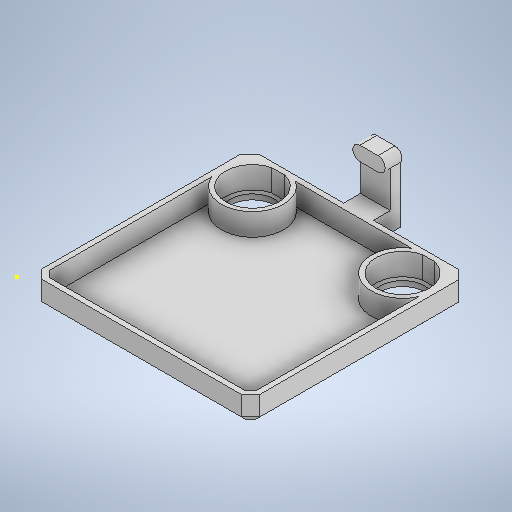
# Autodesk Inventor part: case_v1.4_b
Saved by Autodesk Inventor 2025 (Build 290162000, 162)
## iProperties
Created: 2025-03-20
Part Number: case_v1.4_b
Material: Generic
Document SubType Name: Modeling
Designer: ethan
Density: 1 g/cm^3
Appearance: Default
Author: ethan
Autodesk Inventor part; units mm, degrees
ref_plane "YZ Plane" through (0, 0, 0) normal (1, 0, 0) x (0, 1, 0)
ref_plane "XZ Plane" through (0, 0, 0) normal (0, 1, 0) x (-1, 0, 0)
ref_plane "XY Plane" through (0, 0, 0) normal (0, 0, 1) x (1, 0, 0)
sketch "Sketch1" plane through (0, 0, 0) normal (0, 1, 0) x (-1, 0, 0)
  line L0 (0, 0) -> (-88, 0)
  line L1 (-88, 0) -> (-88, -94)
  line L2 (-88, -94) -> (0, -94)
  line L3 (0, -94) -> (0, 0)
  line L4 (0, -94) -> (0, -75.65)
  line L5 (0, -94) -> (-15.05, -94)
  circle A0 centre (-15.05, -75.65) radius 8.5
  line L6 (-44, -88.9444) -> (-44, -54.2543) construction
  circle A1 centre (-72.95, -75.65) radius 8.5
  line L7 (-15.05, -94) -> (-15.05, -77.2221)
  line L8 (-15.05, -77.2221) -> (-15.05, -73.1555)
  dimension "d0" = 88
  dimension "d1" = 94
  dimension "d2" = 18.35
  dimension "d3" = 15.05
  dimension "d4" = 17
  dimension "d48" = 17
  constraints: 18 end point, 3 point on line, 3 vertical, 2 centre point, 2 parallel, 1 horizontal, 1 perpendicular, 1 symmetric about line, 1 other
  measures "d0" distance of L2.end L1.end
  measures "d1" distance of L1.end L0.end
  measures "d2" distance of L2.end L4.end
  measures "d3" distance of L2.end L5.end
  measures "d4" diameter of A0
  measures "d48" diameter of A1
extrude "Extrusion1" add sketch "Sketch1" along normal blind 2
sketch "Sketch3" plane through (0, 2, 0) normal (0, 1, 0) x (1, 0, 0)
  circle A0 centre (72.95, 75.65) radius 8.5 construction
  circle A1 centre (15.05, 75.65) radius 8.5 construction
  line L0 (0, 0) -> (4, 0) construction
  line L1 (4, 0) -> (4, 6) construction
  line L2 (4, 6) -> (0, 6) construction
  line L3 (0, 6) -> (0, 0) construction
  line L4 (88, 0) -> (84, 0) construction
  line L5 (84, 0) -> (84, 6) construction
  line L6 (84, 6) -> (88, 6) construction
  line L7 (88, 6) -> (88, 0) construction
  line L8 (4, 6) -> (2, 6) construction
  line L9 (2, 6) -> (2, 4) construction
  line L10 (2, 4) -> (4, 4) construction
  line L11 (4, 4) -> (4, 6) construction
  line L12 (2, 4) -> (6, 4)
  line L13 (6, 4) -> (6, 6)
  line L14 (6, 6) -> (2, 6)
  line L15 (2, 6) -> (2, 4)
  line L16 (2, 4) -> (4, 4)
  line L17 (4, 4) -> (4, 8)
  line L18 (4, 8) -> (2, 8)
  line L19 (2, 8) -> (2, 4)
  line L20 (86, 4) -> (82, 4)
  line L21 (82, 4) -> (82, 4)
  line L22 (82, 4) -> (86, 4)
  line L23 (86, 4) -> (86, 4)
  line L24 (86, 4) -> (84, 4)
  line L25 (84, 4) -> (84, 8)
  line L26 (84, 8) -> (86, 8)
  line L27 (86, 8) -> (86, 4)
  line L28 (44, 4.3599) -> (37, 4.3599) construction
  line L29 (88, -1) -> (0, -1) construction
  line L30 (37, -1) -> (51, -1) construction
  line L31 (51, -1) -> (51, 0) construction
  line L32 (51, 0) -> (37, 0) construction
  line L33 (37, 0) -> (37, -1) construction
  line L34 (37, -1) -> (51, -1)
  line L35 (51, -1) -> (51, 0)
  line L36 (51, 0) -> (37, 0)
  line L37 (37, 0) -> (37, -1)
  line L38 (0, 95) -> (88, 95) projected
  line L39 (37, 95) -> (51, 95)
  line L40 (51, 95) -> (51, 94)
  line L41 (51, 94) -> (37, 94)
  line L42 (37, 94) -> (37, 95)
  circle A2 centre (15.05, 75.65) radius 10.5
  circle A3 centre (15.05, 75.65) radius 12
  line L43 (15.05, 75.65) -> (27.05, 75.65) construction
  line L44 (15.05, 75.65) -> (21.05, 86.0423) construction
  line L45 (15.05, 75.65) -> (9.05, 86.0423) construction
  line L46 (15.05, 75.65) -> (3.05, 75.65) construction
  line L47 (15.05, 75.65) -> (9.05, 65.2577) construction
  line L48 (15.05, 75.65) -> (21.05, 65.2577) construction
  line L49 (9.8, 84.7433) -> (9.05, 86.0423) construction
  line L50 (9.8, 84.7433) -> (9.05, 86.0423)
  line L51 (21.05, 86.0423) -> (20.3, 84.7433)
  line L52 (25.55, 75.65) -> (27.05, 75.65)
  line L53 (21.05, 65.2577) -> (20.3, 66.5567)
  line L54 (9.8, 66.5567) -> (9.05, 65.2577)
  line L55 (4.55, 75.65) -> (3.05, 75.65)
  line L56 (44, 84.7433) -> (44, 74.6259) construction
  circle A4 centre (72.95, 75.65) radius 8.5 construction
  circle A5 centre (72.95, 75.65) radius 10.5
  circle A6 centre (72.95, 75.65) radius 12
  line L57 (72.95, 75.65) -> (60.95, 75.65) construction
  line L58 (72.95, 75.65) -> (66.95, 86.0423) construction
  line L59 (72.95, 75.65) -> (78.95, 86.0423) construction
  line L60 (72.95, 75.65) -> (84.95, 75.65) construction
  line L61 (72.95, 75.65) -> (78.95, 65.2577) construction
  line L62 (72.95, 75.65) -> (66.95, 65.2577) construction
  line L63 (78.2, 84.7433) -> (78.95, 86.0423) construction
  line L64 (78.2, 84.7433) -> (78.95, 86.0423)
  line L65 (66.95, 86.0423) -> (67.7, 84.7433)
  line L66 (62.45, 75.65) -> (60.95, 75.65)
  line L67 (66.95, 65.2577) -> (67.7, 66.5567)
  line L68 (78.2, 66.5567) -> (78.95, 65.2577)
  line L69 (83.45, 75.65) -> (84.95, 75.65)
  line L70 (86, 4) -> (82, 4)
  line L71 (82, 4) -> (82, 6)
  line L72 (82, 6) -> (86, 6)
  line L73 (86, 6) -> (86, 4)
  point P0 (2, 4)
  point P1 (4, 6)
  point P2 (84, 4)
  point P3 (84.95, 75.65)
  point P4 (78.95, 65.2577)
  point P5 (3.05, 75.65)
  point P6 (9.05, 65.2577)
  point P7 (84, 6)
  dimension "d11" = 4
  dimension "d12" = 6
  dimension "d13" = 4
  dimension "d14" = 6
  dimension "d15" = 2
  dimension "d16" = 2
  dimension "d17" = 4
  dimension "d18" = 4
  dimension "d19" = 4
  dimension "d20" = 2
  dimension "d21" = 4
  dimension "d22" = 7
  dimension "d23" = 14
  dimension "d24" = 14
  dimension "d25" = 1
  dimension "d26" = 2
  dimension "d27" = 1.5
  dimension "d30" = 360
  constraints: 144 end point, 21 parallel, 19 symmetric about line, 17 point on line, 16 point on circle, 11 perpendicular, 10 horizontal, 7 collinear, 5 centre point, 2 coincident, 1 vertical, 20 other
  measures "d11" distance of L2.end L1.end
  measures "d12" distance of L1.end L0.end
  measures "d13" distance of L5.end L6.end
  measures "d14" distance of L4.end L5.end
  measures "d15" distance of L10.end L9.end
  measures "d16" distance of L9.end L8.end
  measures "d17" distance of L14.end L13.end
  measures "d18" distance of L17.end L16.end
  measures "d19" distance of L21.end L22.end
  measures "d20" distance of L25.end L26.end
  measures "d21" distance of L24.end L25.end
  measures "d22" distance of L28.start L28.end
  measures "d23" distance of L30.start L30.end
  measures "d24" distance of L39.start L39.end
  measures "d25" distance of L39.end L40.end
  measures "d26" radial gap between concentric circles of A1 A2
  measures "d27" radial gap between concentric circles of A2 A3
extrude "Extrusion3" add sketch "Sketch3" along normal blind 8.5 contours L52 A3 L53 A2 | A2 L50 A3 L51 | L54 A3 L55 A2 | L69 A6 L68 A5 | A5 L65 A6 L64 | L67 A6 L66 A5
sketch "Sketch7" plane through (0, 2, 0) normal (0, 1, 0) x (1, 0, 0)
  line L0 (3.05, 75.65) -> (4.55, 75.65) construction
  arc A0 (4.55, 75.65) -> (9.8, 66.5567) centre (15.05, 75.65) ccw construction
  line L1 (9.8, 66.5567) -> (9.05, 65.2577) construction
  arc A1 (3.05, 75.65) -> (9.05, 65.2577) centre (15.05, 75.65) ccw construction
  arc A2 (78.95, 65.2577) -> (84.95, 75.65) centre (72.95, 75.65) ccw construction
  line L2 (78.95, 65.2577) -> (78.2, 66.5567) construction
  arc A3 (78.2, 66.5567) -> (83.45, 75.65) centre (72.95, 75.65) ccw construction
  line L3 (83.45, 75.65) -> (84.95, 75.65) construction
  arc A4 (78.2, 84.7433) -> (67.7, 84.7433) centre (72.95, 75.65) ccw construction
  line L4 (67.7, 84.7433) -> (66.95, 86.0423) construction
  arc A5 (78.95, 86.0423) -> (66.95, 86.0423) centre (72.95, 75.65) ccw construction
  line L5 (78.95, 86.0423) -> (78.2, 84.7433) construction
  line L6 (21.05, 86.0423) -> (20.3, 84.7433) construction
  arc A6 (20.3, 84.7433) -> (9.8, 84.7433) centre (15.05, 75.65) ccw construction
  line L7 (9.8, 84.7433) -> (9.05, 86.0423) construction
  arc A7 (21.05, 86.0423) -> (9.05, 86.0423) centre (15.05, 75.65) ccw construction
  arc A8 (62.45, 75.65) -> (67.7, 66.5567) centre (72.95, 75.65) ccw construction
  line L8 (67.7, 66.5567) -> (66.95, 65.2577) construction
  arc A9 (60.95, 75.65) -> (66.95, 65.2577) centre (72.95, 75.65) ccw construction
  line L9 (60.95, 75.65) -> (62.45, 75.65) construction
  line L10 (25.55, 75.65) -> (27.05, 75.65) construction
  arc A10 (21.05, 65.2577) -> (27.05, 75.65) centre (15.05, 75.65) ccw construction
  line L11 (21.05, 65.2577) -> (20.3, 66.5567) construction
  arc A11 (20.3, 66.5567) -> (25.55, 75.65) centre (15.05, 75.65) ccw construction
  line L12 (88, 94) -> (0, 94) construction
  line L13 (0, 94) -> (0, 0) construction
  line L14 (0, 0) -> (88, 0) construction
  line L15 (88, 0) -> (88, 94) construction
  circle A12 centre (72.95, 75.65) radius 8.5 construction
  circle A13 centre (15.05, 75.65) radius 8.5 construction
  line L16 (2, 4) -> (86, 4) construction
  line L17 (86, 4) -> (86, 94) construction
  line L18 (86, 94) -> (2, 94) construction
  line L19 (2, 94) -> (2, 4) construction
  line L20 (0, 0) -> (88, 0)
  line L21 (88, 0) -> (88, 94)
  line L22 (88, 94) -> (0, 94)
  line L23 (0, 94) -> (0, 0)
  line L24 (86, 94) -> (2, 94)
  line L25 (2, 94) -> (2, 4)
  line L26 (2, 4) -> (86, 4)
  line L27 (86, 4) -> (86, 94)
  point P0 (2, 94)
  constraints: 24 end point, 6 parallel, 3 horizontal, 3 perpendicular, 1 point on line
extrude "Extrusion7" cut sketch "Sketch7" against normal up to surface (2 mm away) contours L23 L22 L25 L26 L27 L21 L20
sketch "Sketch8" plane through (0, 2, 0) normal (0, 1, 0) x (1, 0, 0)
  circle A0 centre (15.05, 75.65) radius 8.5 projected
  circle A1 centre (72.95, 75.65) radius 8.5 projected
  line L0 (86, 4) -> (86, 94) projected
  line L1 (86, 94) -> (2, 94) projected
  line L2 (2, 94) -> (2, 4) projected
  line L3 (3.05, 75.65) -> (4.55, 75.65) projected
  arc A2 (4.55, 75.65) -> (9.8, 66.5567) centre (15.05, 75.65) ccw projected
  line L4 (9.8, 66.5567) -> (9.05, 65.2577) projected
  arc A3 (3.05, 75.65) -> (9.05, 65.2577) centre (15.05, 75.65) ccw projected
  arc A4 (78.95, 65.2577) -> (84.95, 75.65) centre (72.95, 75.65) ccw projected
  line L5 (78.95, 65.2577) -> (78.2, 66.5567) projected
  arc A5 (78.2, 66.5567) -> (83.45, 75.65) centre (72.95, 75.65) ccw projected
  line L6 (83.45, 75.65) -> (84.95, 75.65) projected
  line L7 (25.55, 75.65) -> (27.05, 75.65) projected
  arc A6 (21.05, 65.2577) -> (27.05, 75.65) centre (15.05, 75.65) ccw projected
  line L8 (21.05, 65.2577) -> (20.3, 66.5567) projected
  arc A7 (20.3, 66.5567) -> (25.55, 75.65) centre (15.05, 75.65) ccw projected
  arc A8 (62.45, 75.65) -> (67.7, 66.5567) centre (72.95, 75.65) ccw projected
  line L9 (67.7, 66.5567) -> (66.95, 65.2577) projected
  arc A9 (60.95, 75.65) -> (66.95, 65.2577) centre (72.95, 75.65) ccw projected
  line L10 (60.95, 75.65) -> (62.45, 75.65) projected
  line L11 (21.05, 86.0423) -> (20.3, 84.7433) projected
  arc A10 (20.3, 84.7433) -> (9.8, 84.7433) centre (15.05, 75.65) ccw projected
  line L12 (9.8, 84.7433) -> (9.05, 86.0423) projected
  arc A11 (21.05, 86.0423) -> (9.05, 86.0423) centre (15.05, 75.65) ccw projected
  arc A12 (78.2, 84.7433) -> (67.7, 84.7433) centre (72.95, 75.65) ccw projected
  line L13 (67.7, 84.7433) -> (66.95, 86.0423) projected
  arc A13 (78.95, 86.0423) -> (66.95, 86.0423) centre (72.95, 75.65) ccw projected
  line L14 (78.95, 86.0423) -> (78.2, 84.7433) projected
  line L15 (86, 4) -> (2, 4) projected
  line L16 (2, 75.65) -> (86, 75.65)
  line L17 (86, 75.65) -> (86, 7.5)
  line L18 (82.5, 4) -> (5.5, 4)
  line L19 (2, 7.5) -> (2, 75.65)
  line L20 (2, 7.5) -> (5.5, 4)
  line L21 (82.5, 4) -> (86, 7.5)
  line L22 (4, 73.65) -> (84, 73.65)
  line L23 (84, 73.65) -> (84, 8.3284)
  line L24 (84, 8.3284) -> (81.6716, 6)
  line L25 (81.6716, 6) -> (6.3284, 6)
  line L26 (6.3284, 6) -> (4, 8.3284)
  line L27 (4, 8.3284) -> (4, 73.65)
  line L28 (2, 4) -> (86, 4) projected
  point P0 (0, 0)
  point P1 (2, 4)
  point P2 (4, 70.9705)
  point P3 (3.05, 75.65)
  point P4 (5.5, 4)
  point P5 (84.95, 75.65)
  point P6 (84, 70.9705)
  dimension "d51" = 3.5
  dimension "d52" = 3.5
  dimension "d53" = 3.5
  dimension "d54" = 3.5
  dimension "d55" = 2
  constraints: 24 end point, 4 parallel, 4 point on line, 2 perpendicular, 1 horizontal, 5 other
  measures "d51" distance of L19.start point (2, 4)
  measures "d52" distance of L18.end point (2, 4)
  measures "d53" distance of L18.start L15.start
  measures "d54" distance of L17.end L15.start
  measures "d55" distance between parallel lines of L19 L27
extrude "Extrusion8" add sketch "Sketch8" along normal blind 8.5 contours A3 L27 L26 L25 L24 L23 A4 L16 L0 L21 L15 L20 L2
sketch "Sketch9" plane through (0, 2, 0) normal (0, 1, 0) x (1, 0, 0)
  line L0 (5.5, 4) -> (2, 7.5) projected
  line L1 (2, 7.5) -> (2, 4) projected
  line L2 (2, 4) -> (5.5, 4) projected
  line L3 (86, 4) -> (86, 7.5) projected
  line L4 (86, 7.5) -> (82.5, 4) projected
  line L5 (82.5, 4) -> (86, 4) projected
  line L6 (86, 4) -> (86, 7.5) projected
  line L7 (86, 94) -> (2, 94) projected
  line L8 (5.5, 4) -> (82.5, 4) projected
  line L9 (44, 4) -> (44, 94)
  line L10 (44, 49) -> (73.8977, 49)
  line L11 (5.5, 94) -> (2, 90.5)
  line L12 (2, 90.5) -> (2, 94)
  line L13 (2, 94) -> (5.5, 94)
  line L14 (86, 94) -> (86, 90.5)
  line L15 (86, 90.5) -> (82.5, 94)
  line L16 (82.5, 94) -> (86, 94)
  line L17 (86, 94) -> (86, 90.5)
  line L18 (5.5, 94) -> (82.5, 94)
  point P0 (0, 0)
  point P1 (0, 98)
  constraints: 20 end point, 8 symmetric about line, 3 midpoint, 1 horizontal
extrude "Extrusion9" cut sketch "Sketch9" against normal blind 10 contours L2 L1 L0 | L5 L4 L3
sketch "Sketch10" plane through (0, 2, 0) normal (0, 1, 0) x (1, 0, 0)
  circle A0 centre (15.05, 75.65) radius 8.5 construction
  circle A1 centre (72.95, 75.65) radius 8.5 construction
  line L0 (21.05, 86.0423) -> (20.3, 84.7433) construction
  arc A2 (20.3, 84.7433) -> (9.8, 84.7433) centre (15.05, 75.65) ccw construction
  line L1 (9.8, 84.7433) -> (9.05, 86.0423) construction
  arc A3 (21.05, 86.0423) -> (9.05, 86.0423) centre (15.05, 75.65) ccw construction
  arc A4 (78.2, 84.7433) -> (67.7, 84.7433) centre (72.95, 75.65) ccw construction
  line L2 (67.7, 84.7433) -> (66.95, 86.0423) construction
  arc A5 (78.95, 86.0423) -> (66.95, 86.0423) centre (72.95, 75.65) ccw construction
  line L3 (78.95, 86.0423) -> (78.2, 84.7433) construction
  line L4 (25.55, 75.65) -> (27.05, 75.65) construction
  arc A6 (21.05, 65.2577) -> (27.05, 75.65) centre (15.05, 75.65) ccw construction
  line L5 (21.05, 65.2577) -> (20.3, 66.5567) construction
  arc A7 (20.3, 66.5567) -> (25.55, 75.65) centre (15.05, 75.65) ccw construction
  arc A8 (62.45, 75.65) -> (67.7, 66.5567) centre (72.95, 75.65) ccw construction
  line L6 (67.7, 66.5567) -> (66.95, 65.2577) construction
  arc A9 (60.95, 75.65) -> (66.95, 65.2577) centre (72.95, 75.65) ccw construction
  line L7 (60.95, 75.65) -> (62.45, 75.65) construction
  line L8 (83.45, 75.65) -> (86, 75.65) construction
  line L9 (86, 75.65) -> (86, 94) construction
  line L10 (86, 94) -> (2, 94) construction
  line L11 (2, 94) -> (2, 75.65) construction
  line L12 (2, 75.65) -> (4.55, 75.65) construction
  arc A10 (4.55, 75.65) -> (9.8, 66.5567) centre (15.05, 75.65) ccw construction
  line L13 (9.8, 66.5567) -> (9.05, 65.2577) construction
  arc A11 (4, 70.9705) -> (9.05, 65.2577) centre (15.05, 75.65) ccw construction
  line L14 (4, 70.9705) -> (4, 8.3284) construction
  line L15 (4, 8.3284) -> (6.3284, 6) construction
  line L16 (6.3284, 6) -> (81.6716, 6) construction
  line L17 (81.6716, 6) -> (84, 8.3284) construction
  line L18 (84, 8.3284) -> (84, 70.9705) construction
  arc A12 (78.95, 65.2577) -> (84, 70.9705) centre (72.95, 75.65) ccw construction
  line L19 (78.95, 65.2577) -> (78.2, 66.5567) construction
  arc A13 (78.2, 66.5567) -> (83.45, 75.65) centre (72.95, 75.65) ccw construction
  line L20 (15.05, 87.65) -> (72.95, 87.65) construction
  line L21 (72.95, 87.65) -> (82.5, 87.65) construction
  line L22 (86, 75.65) -> (86, 84.15) construction
  line L23 (82.5, 87.65) -> (86, 84.15) construction
  line L24 (15.05, 87.65) -> (5.5, 87.65) construction
  arc A14 (21.05, 86.0423) -> (9.05, 86.0423) centre (15.05, 75.65) ccw construction
  line L25 (2, 75.65) -> (2, 84.15) construction
  line L26 (5.5, 87.65) -> (2, 84.15) construction
  line L27 (4, 75.65) -> (4, 83.3216) construction
  line L28 (4, 83.3216) -> (6.3284, 85.65) construction
  line L29 (6.3284, 85.65) -> (14.65, 85.65) construction
  line L30 (14.65, 85.65) -> (72.95, 85.65) construction
  line L31 (72.95, 85.65) -> (81.6716, 85.65) construction
  line L32 (81.6716, 85.65) -> (84, 83.3216) construction
  line L33 (84, 83.3216) -> (84, 75.65) construction
  line L34 (2, 75.65) -> (4, 75.65)
  line L35 (4, 75.65) -> (4, 83.3216)
  line L36 (6.3284, 85.65) -> (4, 83.3216)
  line L37 (6.3284, 85.65) -> (81.6716, 85.65)
  line L38 (81.6716, 85.65) -> (84, 83.3216)
  line L39 (84, 83.3216) -> (84, 75.65)
  line L40 (84, 75.65) -> (86, 75.65)
  line L41 (86, 7.5) -> (86, 75.65) projected
  line L42 (86, 75.65) -> (86, 84.15)
  line L43 (86, 84.15) -> (82.5, 87.65)
  line L44 (82.5, 87.65) -> (5.5, 87.65)
  line L45 (5.5, 87.65) -> (2, 84.15)
  line L46 (2, 75.65) -> (2, 84.15)
  point P0 (0, 0)
  point P1 (86, 87.65)
  point P2 (2, 87.65)
  dimension "d60" = 3.5
  dimension "d61" = 3.5
  dimension "d62" = 3.5
  dimension "d63" = 3.5
  dimension "d64" = 2
  constraints: 52 end point, 11 collinear, 7 point on line, 2 perpendicular, 2 point on circle, 1 tangent, 6 other
  measures "d60" distance of L21.end point (86, 87.65)
  measures "d61" distance of L22.end point (86, 87.65)
  measures "d62" distance of L24.end point (2, 87.65)
  measures "d63" distance of L25.end point (2, 87.65)
  measures "d64" distance between parallel lines of L26 L28
extrude "Extrusion10" add sketch "Sketch10" along normal blind 8.5
sketch "Sketch11" plane through (0, 10.5, 0) normal (0, 1, 0) x (1, 0, 0)
  point P0 (0, 0)
sketch "Sketch12" plane through (0, 2, 0) normal (0, 1, 0) x (1, 0, 0)
  line L0 (82.5, 87.65) -> (86, 84.15) projected
  line L1 (86, 84.15) -> (86, 94) projected
  line L2 (86, 94) -> (2, 94) projected
  line L3 (2, 94) -> (2, 84.15) projected
  line L4 (2, 84.15) -> (5.5, 87.65) projected
  line L5 (5.5, 87.65) -> (82.5, 87.65) projected
  point P0 (0, 0)
extrude "Extrusion11" cut sketch "Sketch12" against normal blind 8.5
sketch "Sketch13" plane through (0, 2, 0) normal (0, 1, 0) x (1, 0, 0)
  arc A0 (62.45, 75.65) -> (67.7, 66.5567) centre (72.95, 75.65) ccw projected
  line L0 (67.7, 66.5567) -> (66.95, 65.2577) projected
  arc A1 (60.95, 75.65) -> (66.95, 65.2577) centre (72.95, 75.65) ccw projected
  line L1 (60.95, 75.65) -> (62.45, 75.65) projected
  line L2 (25.55, 75.65) -> (27.05, 75.65) projected
  arc A2 (21.05, 65.2577) -> (27.05, 75.65) centre (15.05, 75.65) ccw projected
  line L3 (21.05, 65.2577) -> (20.3, 66.5567) projected
  arc A3 (20.3, 66.5567) -> (25.55, 75.65) centre (15.05, 75.65) ccw projected
  circle A4 centre (72.95, 75.65) radius 8.5 projected
  circle A5 centre (15.05, 75.65) radius 8.5 projected
  line L4 (76.1516, 85.65) -> (69.7484, 85.65) projected
  arc A6 (69.7484, 85.65) -> (67.7, 84.7433) centre (72.95, 75.65) ccw projected
  line L5 (67.7, 84.7433) -> (67.1765, 85.65) projected
  line L6 (67.1765, 85.65) -> (20.8235, 85.65) projected
  line L7 (20.8235, 85.65) -> (20.3, 84.7433) projected
  arc A7 (20.3, 84.7433) -> (18.2516, 85.65) centre (15.05, 75.65) ccw projected
  line L8 (18.2516, 85.65) -> (11.8484, 85.65) projected
  arc A8 (11.8484, 85.65) -> (9.8, 84.7433) centre (15.05, 75.65) ccw projected
  line L9 (9.8, 84.7433) -> (9.2765, 85.65) projected
  line L10 (9.2765, 85.65) -> (6.3284, 85.65) projected
  line L11 (6.3284, 85.65) -> (4, 83.3216) projected
  line L12 (4, 83.3216) -> (4, 75.65) projected
  line L13 (4, 75.65) -> (4.55, 75.65) projected
  arc A9 (4.55, 75.65) -> (9.8, 66.5567) centre (15.05, 75.65) ccw projected
  line L14 (9.8, 66.5567) -> (9.05, 65.2577) projected
  arc A10 (4, 70.9705) -> (9.05, 65.2577) centre (15.05, 75.65) ccw projected
  line L15 (4, 70.9705) -> (4, 8.3284) projected
  line L16 (4, 8.3284) -> (6.3284, 6) projected
  line L17 (6.3284, 6) -> (81.6716, 6) projected
  line L18 (81.6716, 6) -> (84, 8.3284) projected
  line L19 (84, 8.3284) -> (84, 70.9705) projected
  arc A11 (78.95, 65.2577) -> (84, 70.9705) centre (72.95, 75.65) ccw projected
  line L20 (78.95, 65.2577) -> (78.2, 66.5567) projected
  arc A12 (78.2, 66.5567) -> (83.45, 75.65) centre (72.95, 75.65) ccw projected
  line L21 (83.45, 75.65) -> (84, 75.65) projected
  line L22 (84, 75.65) -> (84, 83.3216) projected
  line L23 (84, 83.3216) -> (81.6716, 85.65) projected
  line L24 (81.6716, 85.65) -> (78.7235, 85.65) projected
  line L25 (78.7235, 85.65) -> (78.2, 84.7433) projected
  arc A13 (78.2, 84.7433) -> (76.1516, 85.65) centre (72.95, 75.65) ccw projected
  circle A14 centre (15.05, 75.65) radius 10.3149
  circle A15 centre (15.05, 75.65) radius 11.75
  circle A16 centre (72.95, 75.65) radius 10.25
  circle A17 centre (72.95, 75.65) radius 11.75
  point P0 (0, 0)
  point P1 (8.8805, 85.65)
  point P2 (4, 79.645)
  point P3 (4.7351, 75.65)
  point P4 (9.8926, 84.5829)
  point P5 (9.175, 65.4742)
  point P6 (20.925, 65.4742)
  point P7 (20.2074, 66.7171)
  point P8 (9.8926, 66.7171)
  point P9 (26.8, 75.65)
  point P10 (21.2195, 85.65)
  point P11 (20.2074, 84.5829)
  point P12 (25.3649, 75.65)
  point P13 (67.075, 65.4742)
  point P14 (78.825, 65.4742)
  point P15 (78.075, 66.7732)
  point P16 (67.825, 66.7732)
  point P17 (83.2, 75.65)
  point P18 (84, 79.645)
  point P19 (79.1195, 85.65)
  point P20 (78.075, 84.5268)
  point P21 (66.7805, 85.65)
  point P22 (61.2, 75.65)
  point P23 (62.7, 75.65)
  point P24 (67.825, 84.5268)
  point P25 (12.5209, 85.65)
  point P26 (17.5791, 85.65)
  point P27 (70.7, 85.65)
  point P28 (75.2, 85.65)
  constraints: 4 centre point
extrude "Extrusion12" add sketch "Sketch13" along normal blind 8.5 contours L1 A17 L6 L5 A6 L4 A16 A13 L25 L24 L22 L21 A12 L20 L0 A0 | A0 L0 A17 L1 | A17 L0 A1 L1 | A17 L24 L25 A13 L4 A16 A6 L5 L6 | L20 A12 L21 L22 A17 | A15 L2 A3 L3 L14 A9 L13 L12 L10 L9 A8 L8 A14 A7 L7 L6 | L6 L7 A7 L8 A14 A8 L9 L10 A15 | L24 L23 L22 A17 | A15 L3 A3 L2 | L2 A2 L3 A15 | A15 L12 L11 L10 | L12 L13 A9 L14 A15 | A16 L4 | L8 A14 picked at (73.2018, 85.724) picked at (15.3336, 85.7433)
sketch "Sketch14" plane through (82.5, 10.5, -87.65) normal (0, 0, -1) x (-1, 0, 0)
  line L0 (0, 0) -> (77, 0) construction
  line L1 (0, 0) -> (0, -10.5) construction
  line L2 (77, -10.5) -> (0, -10.5) construction
  line L3 (77, 0) -> (77, -10.5) construction
  line L4 (44.25, -21) -> (32.75, -21) construction
  line L5 (32.75, -21) -> (32.75, 0) construction
  line L6 (32.75, 0) -> (44.25, 0) construction
  line L7 (44.25, 0) -> (44.25, -21) construction
  line L8 (44.25, -21) -> (32.75, 0) construction
  line L9 (32.75, -21) -> (44.25, 0) construction
  line L10 (44.25, -10.5) -> (32.75, -10.5) construction
  line L11 (32.75, 13.5) -> (32.75, 13.5) construction
  line L12 (32.75, 13.5) -> (44.25, 13.5) construction
  line L13 (44.25, 13.5) -> (44.25, 13.5) construction
  line L14 (42, 15.75) -> (35, 15.75) construction
  line L15 (32.75, 13.5) -> (32.75, 11.25) construction
  line L16 (35, 11.25) -> (42, 11.25) construction
  line L17 (44.25, 11.25) -> (44.25, 13.5) construction
  line L18 (44.25, 15.75) -> (32.75, 11.25) construction
  line L19 (32.75, 15.75) -> (44.25, 11.25) construction
  arc A0 (44.25, 13.5) -> (42, 15.75) centre (42, 13.5) ccw construction
  arc A1 (42, 11.25) -> (44.25, 13.5) centre (42, 13.5) ccw construction
  arc A2 (32.75, 13.5) -> (35, 11.25) centre (35, 13.5) ccw construction
  arc A3 (35, 15.75) -> (32.75, 13.5) centre (35, 13.5) ccw construction
  line L20 (44.25, 0) -> (32.75, 0)
  line L21 (32.75, 0) -> (32.75, -10.5)
  line L22 (32.75, -10.5) -> (44.25, -10.5)
  line L23 (44.25, -10.5) -> (44.25, 0)
  point P0 (82.5, -10.5)
  point P1 (38.5, -10.5)
  point P2 (38.5, 13.5)
  dimension "d71" = 11.5
  dimension "d72" = 24
  dimension "d73" = 4.5
  dimension "d74" = 2.25
  constraints: 40 end point, 9 parallel, 8 point on circle, 8 point on line, 8 tangent, 7 midpoint, 4 centre point, 4 perpendicular, 3 equal radius, 2 horizontal
  measures "d71" distance of L4.start L4.end
  measures "d72" distance of L10.end L11.end
  measures "d73" distance of L15.end L19.start
  measures "d74" radius of A0
extrude "Extrusion13" add sketch "Sketch14" along normal blind 6.5
sketch "Sketch15" plane through (82.5, 10.5, -94.15) normal (0, 0, -1) x (-1, 0, 0)
  line L0 (32.75, -10.5) -> (44.25, -10.5) projected
  line L1 (44.25, -10.5) -> (32.75, -10.5)
  line L2 (32.75, -10.5) -> (32.75, 15.75)
  line L3 (32.75, 15.75) -> (44.25, 15.75)
  line L4 (44.25, 15.75) -> (44.25, -10.5)
  line L5 (42, 18) -> (35, 18)
  line L6 (32.75, 15.75) -> (32.75, 13.5)
  line L7 (32.75, 13.5) -> (44.25, 13.5)
  line L8 (44.25, 13.5) -> (44.25, 15.75)
  line L9 (44.25, 18) -> (32.75, 13.5) construction
  line L10 (32.75, 18) -> (44.25, 13.5) construction
  arc A0 (44.25, 15.75) -> (42, 18) centre (42, 15.75) ccw
  arc A1 (35, 18) -> (32.75, 15.75) centre (35, 15.75) ccw
  point P0 (82.5, -10.5)
  point P1 (38.5, 15.75)
  point P2 (44.25, 15.75)
  dimension "d77" = 11.5
  dimension "d78" = 26.25
  dimension "d79" = 4.5
  dimension "d80" = 2.25
  constraints: 20 end point, 5 parallel, 4 point on circle, 4 point on line, 4 tangent, 3 midpoint, 2 centre point, 2 perpendicular, 1 equal radius, 1 horizontal
  measures "d77" distance of L2.end L3.end
  measures "d78" distance of L1.end L2.end
  measures "d79" distance of L6.end L10.start
  measures "d80" radius of A0
extrude "Extrusion14" add sketch "Sketch15" along normal blind 2
sketch "Sketch16" plane through (82.5, 10.5, -94.15) normal (0, 0, 1) x (1, 0, 0)
  line L0 (-44.25, 0) -> (-32.75, 0) construction
  line L1 (-32.75, 15.75) -> (-32.75, 0) construction
  arc A0 (-32.75, 15.75) -> (-35, 18) centre (-35, 15.75) ccw construction
  line L2 (-42, 18) -> (-35, 18) construction
  arc A1 (-42, 18) -> (-44.25, 15.75) centre (-42, 15.75) ccw construction
  line L3 (-44.25, 0) -> (-44.25, 15.75) construction
  circle A2 centre (-35, 15.75) radius 2.25 construction
  circle A3 centre (-42, 15.75) radius 2.25 construction
  line L4 (-35, 13.5) -> (-42, 13.5) construction
  line L5 (-35, 13.5) -> (-42, 13.5)
  line L6 (-42, 18) -> (-35, 18)
  arc A4 (-32.75, 15.75) -> (-35, 18) centre (-35, 15.75) ccw projected
  arc A5 (-35, 13.5) -> (-35, 18) centre (-35, 15.75) ccw
  arc A6 (-42, 18) -> (-42, 13.5) centre (-42, 15.75) ccw
  point P0 (-82.5, -10.5)
  constraints: 11 point on circle, 8 tangent, 6 end point, 4 centre point, 2 coincident, 1 collinear, 1 point on line
extrude "Extrusion15" add sketch "Sketch16" along normal blind 2.5
chamfer "Chamfer1" distance 3 angle 45 9 edges at (2, 0, -45.825) (3.75, 0, -85.9) (21.875, 0, -87.65) (66.125, 0, -87.65) (84.25, 0, -85.9) (86, 0, -45.825) (44, 0, -4) (84.25, 0, -5.75) (3.75, 0, -5.75)
sketch "Sketch17" plane through (82.5, 10.5, -96.15) normal (0, 0, -1) x (-1, 0, 0)
  line L0 (32.75, -10.5) -> (44.25, -10.5) construction
  line L1 (44.25, -10.5) -> (44.25, 15.75) construction
  arc A0 (44.25, 15.75) -> (42, 18) centre (42, 15.75) ccw construction
  line L2 (42, 18) -> (35, 18) construction
  arc A1 (35, 18) -> (32.75, 15.75) centre (35, 15.75) ccw construction
  line L3 (32.75, 15.75) -> (32.75, -10.5) construction
  arc A2 (44.75, 15.75) -> (42, 18.5) centre (42, 15.75) ccw construction
  line L4 (44.75, 15.75) -> (44.75, -11) construction
  line L5 (44.75, -11) -> (32.25, -11) construction
  line L6 (32.25, -11) -> (32.25, 15.75) construction
  arc A3 (35, 18.5) -> (32.25, 15.75) centre (35, 15.75) ccw construction
  line L7 (35, 18.5) -> (42, 18.5) construction
  circle A4 centre (42, 15.75) radius 2.75 construction
  circle A5 centre (35, 15.75) radius 2.75 construction
  line L8 (42, 13) -> (35, 13)
  line L9 (35, 18.5) -> (42, 18.5)
  arc A6 (42, 13) -> (42, 18.5) centre (42, 15.75) ccw
  arc A7 (35, 18.5) -> (35, 13) centre (35, 15.75) ccw
  point P0 (82.5, -10.5)
  dimension "d88" = 0.5
  constraints: 12 end point, 8 point on circle, 4 centre point, 3 horizontal, 3 tangent, 2 coincident, 2 vertical alignment, 1 parallel, 1 perpendicular, 9 other
  measures "d88" radial gap between concentric circles of A0 A2
extrude "Extrusion16" add sketch "Sketch17" against normal up to surface (4.5 mm away)
sketch "Sketch18" plane through (82.5, 10.5, -96.15) normal (0, 0, -1) x (-1, 0, 0)
  arc A0 (44.25, 14.1689) -> (42, 18.5) centre (42, 15.75) ccw projected
  line L0 (42, 18.5) -> (35, 18.5) projected
  arc A1 (35, 18.5) -> (32.75, 14.1689) centre (35, 15.75) ccw projected
  line L1 (32.75, 14.1689) -> (32.75, -10.5) projected
  line L2 (32.75, -10.5) -> (44.25, -10.5) projected
  line L3 (44.25, -10.5) -> (44.25, 14.1689) projected
  point P0 (82.5, -10.5)
extrude "Extrusion17" add sketch "Sketch18" along normal blind 2
chamfer "Chamfer2" distance 3 angle 45 4 edges at (38.25, 0, -97.15) (38.25, 0, -90.4) (44, 0, -98.15) (49.75, 0, -90.4)
sketch "Sketch19" plane through (0, 2, 0) normal (0, 1, 0) x (1, 0, 0)
  arc A0 (9.175, 65.4742) -> (20.925, 65.4742) centre (15.05, 75.65) ccw projected
  line L0 (9.175, 65.4742) -> (9.05, 65.2577) projected
  arc A1 (4, 70.9705) -> (9.05, 65.2577) centre (15.05, 75.65) ccw projected
  line L1 (4, 70.9705) -> (4, 8.3284) projected
  line L2 (4, 8.3284) -> (6.3284, 6) projected
  line L3 (6.3284, 6) -> (81.6716, 6) projected
  line L4 (81.6716, 6) -> (84, 8.3284) projected
  line L5 (84, 8.3284) -> (84, 70.9705) projected
  arc A2 (78.95, 65.2577) -> (84, 70.9705) centre (72.95, 75.65) ccw projected
  line L6 (78.95, 65.2577) -> (78.825, 65.4742) projected
  arc A3 (67.075, 65.4742) -> (78.825, 65.4742) centre (72.95, 75.65) ccw projected
  line L7 (67.075, 65.4742) -> (66.95, 65.2577) projected
  arc A4 (60.95, 75.65) -> (66.95, 65.2577) centre (72.95, 75.65) ccw projected
  line L8 (60.95, 75.65) -> (61.2, 75.65) projected
  arc A5 (66.7805, 85.65) -> (61.2, 75.65) centre (72.95, 75.65) ccw projected
  line L9 (66.7805, 85.65) -> (21.2195, 85.65) projected
  arc A6 (26.8, 75.65) -> (21.2195, 85.65) centre (15.05, 75.65) ccw projected
  line L10 (26.8, 75.65) -> (27.05, 75.65) projected
  arc A7 (21.05, 65.2577) -> (27.05, 75.65) centre (15.05, 75.65) ccw projected
  line L11 (21.05, 65.2577) -> (20.925, 65.4742) projected
  arc A8 (21.05, 65.2577) -> (27.05, 75.65) centre (15.05, 75.65) ccw projected
  circle A9 centre (15.05, 75.65) radius 12
  circle A10 centre (72.95, 75.65) radius 12
  circle A11 centre (72.95, 75.65) radius 10.2605
  circle A12 centre (15.05, 75.65) radius 8.5
  line L12 (67.979, 86.572) -> (77.921, 86.572)
  line L13 (20.021, 86.572) -> (10.079, 86.572)
  point P0 (0, 0)
  point P1 (66.3168, 85.65)
  point P2 (21.6832, 85.65)
  constraints: 6 point on circle, 4 centre point, 4 end point, 3 coincident, 1 horizontal
extrude "Extrusion18" add sketch "Sketch19" along normal blind 8.5 contours A0 L11 A9 L0 | L10 A6 L9 A9 | L9 A5 L8 A10 | L7 A3 L6 A10
equation "\"d52\" = d51"
equation "\"d53\" = d51"
equation "\"d54\" = d53"
equation "\"d61\" = d60"
equation "\"d63\" = d62"
body "Solid1"
